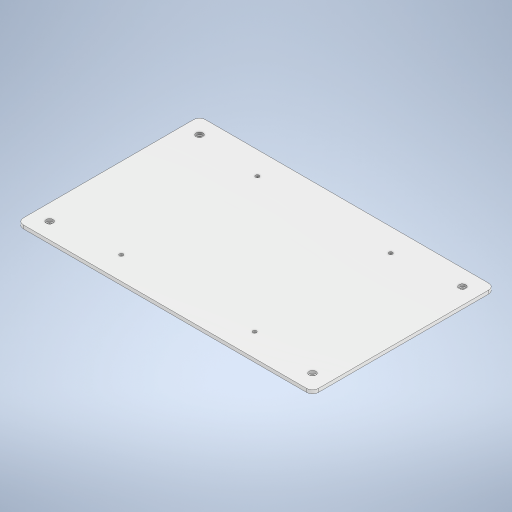
# Autodesk Inventor part: BP_BOX-Above
Saved by Autodesk Inventor 2024.3 (Build 283343000, 343)
## iProperties
Created: 2025-04-29
Part Number: BP_BOX-Above
Material: アセタール樹脂、白
Document SubType Name: Modeling
Designer: ngt-a
Density: 1.425 g/cm^3
Appearance: 滑らか - 白
Mass: 180.144 g
Surface Area: 870.17 cm^2
Volume: 126.417 cm^3
Author: ngt-a
Autodesk Inventor part; units mm, degrees
ref_plane "YZ Plane" through (0, 0, 0) normal (1, 0, 0) x (0, 1, 0)
ref_plane "XZ Plane" through (0, 0, 0) normal (0, 1, 0) x (-1, 0, 0)
ref_plane "XY Plane" through (0, 0, 0) normal (0, 0, 1) x (1, 0, 0)
sketch "スケッチ1" plane through (0, 0, 0) normal (0, 1, 0) x (-1, 0, 0)
  line L0 (130, 81) -> (-130, 81)
  line L1 (-130, 81) -> (-130, -81)
  line L2 (-130, -81) -> (130, -81)
  line L3 (130, -81) -> (130, 81)
  line L4 (130, 81) -> (-130, -81) construction
  line L5 (-130, 81) -> (130, -81) construction
  point P0 (0, 0)
  dimension "d0" = 260
  dimension "d1" = 162
  constraints: 12 end point, 2 midpoint, 2 parallel, 1 horizontal, 1 perpendicular
  measures "d0" distance of L1.end L2.end
  measures "d1" distance of L2.end L0.start
extrude "押し出し1" add sketch "スケッチ1" along normal blind 3
sketch "スケッチ7" plane through (0, 3, 0) normal (0, 1, 0) x (1, 0, 0)
  line L0 (-130, 81) -> (-130, -81) projected
  line L1 (130, -81) -> (130, 81) projected
  line L2 (130, 81) -> (-130, 81) projected
  point P0 (0, 0)
  point P1 (-116, 67)
  point P2 (112, 67)
  point P3 (112, -63)
  point P4 (-116, -63)
  dimension "d23" = 14
  dimension "d25" = 130
  dimension "d26" = 130
  dimension "d27" = 14
  dimension "d29" = 14
  dimension "d38" = 228
  dimension "d39" = 228
  dimension "d40" = 14
  measures "d23" distance from line of L0 point (-116, 67)
  measures "d25" distance of point (112, -63) point (112, 67)
  measures "d26" distance of point (-116, -63) point (-116, 67)
  measures "d27" distance from line of L0 point (-116, -63)
  measures "d29" distance from line of L2 point (-116, 67)
  measures "d38" distance of point (-116, -63) point (112, -63)
  measures "d39" distance of point (-116, 67) point (112, 67)
  measures "d40" distance from line of L2 point (112, 67)
hole "穴1" at (-116, 3, -67) at (112, 3, -67) at (112, 3, 63) at (-116, 3, 63) direction (0, -1, 0) diameter 3.2 depth 8
sketch "スケッチ8" plane through (0, 3, 0) normal (0, 1, 0) x (1, 0, 0)
  line L0 (130, 81) -> (-130, 81) projected
  line L1 (-130, 81) -> (126, 81)
  line L2 (126, 81) -> (126, -77)
  line L3 (126, -77) -> (-130, -77)
  line L4 (-130, -77) -> (-130, 81)
  circle A0 centre (-116, 67) radius 1.6 projected
  circle A1 centre (112, 67) radius 1.6 projected
  circle A2 centre (-116, -63) radius 1.6 projected
  circle A3 centre (-116, -63) radius 1.6 projected
  circle A4 centre (112, -63) radius 1.6 projected
  circle A5 centre (112, 67) radius 1.6 projected
  circle A6 centre (-116, 67) radius 1.6 projected
  line L5 (130, -81) -> (130, 81) projected
  line L6 (130, 81) -> (-130, 81) projected
  line L7 (-130, 81) -> (-130, -81) projected
  line L8 (-130, -81) -> (130, -81) projected
  point P0 (0, 0)
  dimension "d41" = 14
  dimension "d42" = 14
  dimension "d43" = 14
  constraints: 8 end point, 2 parallel, 1 horizontal, 1 perpendicular
  measures "d41" distance from line of L4 A0.centre
  measures "d42" distance from line of L2 A1.centre
  measures "d43" distance from line of L3 A2.centre
extrude "押し出し4" cut sketch "スケッチ8" against normal blind 10 contours L5 L8 L7 L3 L2 L0
fillet "フィレット1" radius 5 4 edges at (-130, 1.5, -81) (-130, 1.5, 77) (126, 1.5, -81) (126, 1.5, 77)
sketch "スケッチ9" plane through (0, 3, 0) normal (0, 1, 0) x (1, 0, 0)
  arc A0 (121, -77) -> (126, -72) centre (121, -72) ccw projected
  line L0 (126, -72) -> (126, 76) projected
  arc A1 (126, 76) -> (121, 81) centre (121, 76) ccw projected
  line L1 (121, 81) -> (-125, 81) projected
  arc A2 (-125, 81) -> (-130, 76) centre (-125, 76) ccw projected
  line L2 (-130, 76) -> (-130, -72) projected
  arc A3 (-130, -72) -> (-125, -77) centre (-125, -72) ccw projected
  line L3 (-125, -77) -> (121, -77) projected
  circle A4 centre (-116, 67) radius 1.6 projected
  circle A5 centre (112, 67) radius 1.6 projected
  circle A6 centre (112, -63) radius 1.6 projected
  circle A7 centre (-116, -63) radius 1.6 projected
  circle A8 centre (-116, 67) radius 3
  circle A9 centre (-116, -63) radius 3
  circle A10 centre (112, -63) radius 3
  circle A11 centre (112, 67) radius 3
  point P0 (0, 0)
  dimension "d47" = 6
  dimension "d48" = 6
  dimension "d49" = 6
  dimension "d50" = 6
  constraints: 4 centre point
  measures "d47" diameter of A8
  measures "d48" diameter of A9
  measures "d49" diameter of A10
  measures "d50" diameter of A11
extrude "押し出し5" cut sketch "スケッチ9" against normal blind 2 contours A4 | A5 | A6 | A7 | A8 | A9 | A10 | A11
sketch "スケッチ10" plane through (0, 3, 0) normal (0, 1, 0) x (1, 0, 0)
  line L0 (121, 81) -> (-125, 81) projected
  line L1 (121, -77) -> (-125, -77) projected
  line L2 (-90, 81) -> (-69.8, 81)
  line L3 (-69.8, 81) -> (-69.8, -77)
  line L4 (-69.8, -77) -> (-90, -77)
  line L5 (-90, -77) -> (-90, 81)
  line L6 (86, 81) -> (65.8, 81)
  line L7 (65.8, 81) -> (65.8, -77)
  line L8 (65.8, -77) -> (86, -77)
  line L9 (86, -77) -> (86, 81)
  line L10 (-69.8, 81) -> (-49.6, 81)
  line L11 (-49.6, 81) -> (-49.6, -77)
  line L12 (-49.6, -77) -> (-69.8, -77)
  line L13 (-69.8, -77) -> (-69.8, 81)
  line L14 (65.8, 81) -> (45.6, 81)
  line L15 (45.6, 81) -> (45.6, -77)
  line L16 (45.6, -77) -> (65.8, -77)
  line L17 (65.8, -77) -> (65.8, 81)
  line L18 (45.6, -77) -> (25.4, -77)
  line L19 (25.4, -77) -> (25.4, 81)
  line L20 (25.4, 81) -> (45.6, 81)
  line L21 (45.6, 81) -> (45.6, -77)
  line L22 (-49.6, 81) -> (-29.4, 81)
  line L23 (-29.4, 81) -> (-29.4, -77)
  line L24 (-29.4, -77) -> (-49.6, -77)
  line L25 (-49.6, -77) -> (-49.6, 81)
  line L26 (-130, 76) -> (-130, -72) projected
  line L27 (126, -72) -> (126, 76) projected
  line L28 (-69.7, 81) -> (-49.7, 81)
  line L29 (-49.7, 81) -> (-49.7, -77)
  line L30 (-49.7, -77) -> (-69.7, -77)
  line L31 (-69.7, -77) -> (-69.7, 81)
  line L32 (0, 0) -> (0, 23.1289)
  line L33 (-69.9, 81) -> (-87.9535, 81)
  line L34 (-87.9535, 81) -> (-87.9535, -77)
  line L35 (-87.9535, -77) -> (-69.9, -77)
  line L36 (-69.9, -77) -> (-69.9, 81)
  point P0 (-59.8, 61)
  point P1 (-59.8, -57)
  point P2 (55.8, 61)
  point P3 (55.8, -57)
  dimension "d53" = 20.2
  dimension "d54" = 20.2
  dimension "d55" = 20.2
  dimension "d56" = 20.2
  dimension "d57" = 20.2
  dimension "d58" = 20.2
  dimension "d59" = 40
  dimension "d60" = 40
  dimension "d61" = 0.1
  dimension "d62" = 0.1
  dimension "d63" = 20
  dimension "d64" = 20
  dimension "d66" = 256
  dimension "d67" = 158
  dimension "d68" = 0.2
  dimension "d69" = 20
  dimension "d70" = 118
  dimension "d71" = 70.2
  dimension "d72" = 70.2
  dimension "d80" = 70.2
  dimension "d81" = 70.2
  dimension "d14" = 30
  dimension "d15" = 30
  dimension "d16" = 30
  dimension "d17" = 30
  constraints: 66 end point, 16 parallel, 12 point on line, 8 horizontal, 8 perpendicular, 1 vertical
  measures "d53" distance between parallel lines of L11 L3
  measures "d54" distance between parallel lines of L23 L25
  measures "d55" distance between parallel lines of L5 L3
  measures "d56" distance between parallel lines of L19 L15
  measures "d57" distance between parallel lines of L15 L7
  measures "d58" distance between parallel lines of L7 L9
  measures "d59" distance between parallel lines of L26 L5
  measures "d60" distance between parallel lines of L27 L9
  measures "d61" distance between parallel lines of L11 L29
  measures "d62" distance between parallel lines of L3 L31
  measures "d63" distance from line of L0 point (-59.8, 61)
  measures "d64" distance from line of L1 point (-59.8, -57)
  measures "d66" distance between parallel lines of L27 L26
  measures "d67" distance between parallel lines of L1 L0
  measures "d68" distance between parallel lines of L31 L36
  measures "d69" distance from line of L16 point (55.8, -57)
  measures "d70" distance of point (55.8, -57) point (55.8, 61)
  measures "d71" distance from line of L27 point (55.8, 61)
  measures "d72" distance from line of L27 point (55.8, -57)
  measures "d80" distance from line of L26 point (-59.8, 61)
  measures "d81" distance from line of L26 point (-59.8, -57)
hole "穴2" at (-59.8, 3, -61) at (-59.8, 3, 57) at (55.8, 3, -61) at (55.8, 3, 57) direction (0, -1, 0) diameter 3.2 depth 8
equation "\"d26\" = d25"
equation "\"d27\" = d23"
equation "\"d39\" = d38"
equation "\"d42\" = d41"
equation "\"d43\" = d41"
equation "\"d48\" = d47"
equation "\"d49\" = d47"
equation "\"d50\" = d47"
equation "\"d54\" = d53"
equation "\"d55\" = d53"
equation "\"d56\" = d54"
equation "\"d57\" = d56"
equation "\"d58\" = d57"
equation "\"d62\" = d61"
equation "\"d64\" = d63"
equation "\"d71\" = d72"
equation "\"d81\" = d80"
